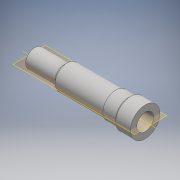
# Autodesk Inventor part: Полый вал
Saved by Autodesk Inventor 2016 SP1 (Build 200210100, 210)
## iProperties
Created: 2016-05-02
Part Number: Полый вал
Material: Типовые
Document SubType Name: Modeling
Designer: AS
Density: 1 g/cm^3
Appearance: По умолчанию
Author: AS
Autodesk Inventor part; units mm, degrees
ref_plane "YZ Plane" through (0, 0, 0) normal (1, 0, 0) x (0, 1, 0)
ref_plane "XZ Plane" through (0, 0, 0) normal (0, 1, 0) x (-1, 0, 0)
sketch "Эскиз1" plane through (0, 0, 0) normal (0, 0, 1) x (1, 0, 0)
  line L0 (153.4512, -23) -> (-146.5488, -23)
  line L1 (153.4512, -23) -> (153.4512, -40)
  line L2 (153.4512, -40) -> (108.4512, -40)
  line L3 (108.4512, -40) -> (108.4512, -35)
  line L4 (108.4512, -35) -> (73.4512, -35)
  line L5 (73.4512, -35) -> (73.4512, -33)
  line L6 (73.4512, -33) -> (-66.5488, -33)
  line L7 (-66.5488, -33) -> (-66.5488, -25)
  line L8 (-66.5488, -25) -> (-146.5488, -25)
  line L9 (-146.5488, -25) -> (-146.5488, -23)
  line L10 (-206.5488, 0) -> (213.4512, 0) projected
  point P0 (0, 0)
  dimension "d0" = 300
  dimension "d1" = 17
  dimension "d2" = 2
  dimension "d3" = 10
  dimension "d4" = 12
  dimension "d5" = 80
  dimension "d6" = 140
  dimension "d7" = 35
  dimension "d8" = 45
  dimension "d10" = 23
  constraints: 20 end point, 8 perpendicular, 1 horizontal, 1 vertical
  measures "d0" distance of L0.start L0.end
  measures "d1" distance between parallel lines of L2 L0
  measures "d2" distance between parallel lines of L8 L0
  measures "d3" distance between parallel lines of L6 L0
  measures "d4" distance between parallel lines of L4 L0
  measures "d5" distance between parallel lines of L7 L9
  measures "d6" distance between parallel lines of L7 L5
  measures "d7" distance from line of L3.end L5
  measures "d8" distance between parallel lines of L1 L3
  measures "d10" distance between parallel lines of L0 L10
revolve "Вращение1" add sketch "Эскиз1" angle 360 about axis through (-10, 0, 0) along (1, 0, 0)
chamfer "Фаска1" distance 5 angle 45 1 edges at (108.4512, 40, 0)
chamfer "Фаска2" distance 8 angle 45 1 edges at (-66.5488, 33, 0)
